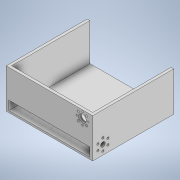
# Autodesk Inventor part: Box
Saved by Autodesk Inventor 2020.3 (Build 243373010, 373A)
## iProperties
Created: 2020-12-16
Part Number: Box
Material: Generic
Document SubType Name: Modeling
Designer: Owner
Density: 1 g/cm^3
Appearance: Default
Author: Owner
Autodesk Inventor part; units mm, degrees
ref_plane "YZ Plane" through (0, 0, 0) normal (1, 0, 0) x (0, 1, 0)
ref_plane "XZ Plane" through (0, 0, 0) normal (0, 1, 0) x (-1, 0, 0)
ref_plane "XY Plane" through (0, 0, 0) normal (0, 0, 1) x (1, 0, 0)
sketch "Sketch1" plane through (0, 0, 0) normal (0, 1, 0) x (-1, 0, 0)
  line L0 (73.3806, 68.834) -> (-73.3806, 68.834)
  line L1 (-73.3806, 68.834) -> (-73.3806, -68.834)
  line L2 (-73.3806, -68.834) -> (73.3806, -68.834)
  line L3 (73.3806, -68.834) -> (73.3806, 68.834)
  line L4 (73.3806, 68.834) -> (-73.3806, -68.834) construction
  line L5 (-73.3806, 68.834) -> (73.3806, -68.834) construction
  point P0 (0, 0)
  dimension "d0" = 146.7612
  dimension "d1" = 137.668
  constraints: 12 end point, 2 midpoint, 2 parallel, 1 horizontal, 1 perpendicular
  measures "d0" distance of L2.end L1.end
  measures "d1" distance of L1.end L0.end
extrude "Extrusion1" add sketch "Sketch1" along normal blind 3.175
sketch "Sketch2" plane through (0, 3.175, 0) normal (0, 1, 0) x (1, 0, 0)
  line L0 (73.3806, 68.834) -> (-73.3806, 68.834) projected
  line L1 (-68.834, -68.834) -> (68.834, -68.834)
  line L2 (68.834, -68.834) -> (68.834, 68.834)
  line L3 (68.834, 68.834) -> (-68.834, 68.834)
  line L4 (-68.834, 68.834) -> (-68.834, -68.834)
  line L5 (-68.834, -68.834) -> (68.834, 68.834) construction
  line L6 (68.834, -68.834) -> (-68.834, 68.834) construction
  line L7 (73.3806, -68.834) -> (73.3806, 68.834) projected
  line L8 (73.3806, 68.834) -> (68.834, 68.834)
  line L9 (68.834, 68.834) -> (68.834, -68.834)
  line L10 (68.834, -68.834) -> (73.3806, -68.834)
  line L11 (73.3806, -68.834) -> (73.3806, 68.834)
  line L12 (-73.3806, 68.834) -> (-68.834, 68.834)
  line L13 (-68.834, 68.834) -> (-68.834, -68.834)
  line L14 (-68.834, -68.834) -> (-73.3806, -68.834)
  line L15 (-73.3806, -68.834) -> (-73.3806, 68.834)
  point P0 (0, 0)
  dimension "d4" = 137.668
  constraints: 28 end point, 6 parallel, 3 horizontal, 3 perpendicular, 2 midpoint, 1 point on line
  measures "d4" distance of L3.end L2.end
extrude "Extrusion2" add sketch "Sketch2" along normal blind 63.5 contours L7 L10 L2 L0 | L4 L14 L15 L0
sketch "Sketch3" plane through (0, 3.175, 0) normal (0, 1, 0) x (1, 0, 0)
  line L0 (-68.834, -68.834) -> (68.834, -68.834) projected
  line L1 (68.834, 68.834) -> (68.834, -68.834) projected
  line L2 (-68.834, -68.834) -> (68.834, -68.834)
  line L3 (68.834, -68.834) -> (68.834, -64.2874)
  line L4 (68.834, -64.2874) -> (-68.834, -64.2874)
  line L5 (-68.834, -64.2874) -> (-68.834, -68.834)
  point P0 (0, 0)
  dimension "d7" = 4.5466
  constraints: 8 end point, 2 parallel, 1 horizontal, 1 perpendicular, 1 point on line
  measures "d7" distance of L3.end L2.end
extrude "Extrusion3" add sketch "Sketch3" along normal blind 63.5
sketch "Sketch4" plane through (-73.3806, 0, 68.834) normal (0, 0, 1) x (1, 0, 0)
  line L0 (142.2146, 3.175) -> (4.5466, 3.175) projected
  line L1 (142.2146, 3.175) -> (142.2146, 66.675) projected
  line L2 (4.5466, 3.175) -> (142.2146, 3.175)
  line L3 (142.2146, 3.175) -> (142.2146, 18.415)
  line L4 (142.2146, 18.415) -> (4.5466, 18.415)
  line L5 (4.5466, 18.415) -> (4.5466, 3.175)
  point P0 (73.3806, 0)
  dimension "d10" = 15.24
  constraints: 8 end point, 2 parallel, 1 horizontal, 1 perpendicular, 1 point on line
  measures "d10" distance of L3.end L2.end
extrude "Extrusion4" cut sketch "Sketch4" against normal blind 25.4
sketch "Sketch5" plane through (73.3806, 0, 68.834) normal (1, 0, 0) x (0, 0, -1)
  line L0 (4.5466, 66.675) -> (4.5466, 18.415) projected
  line L1 (4.5466, 20.7271) -> (4.5466, 3.175)
  line L2 (0, 3.175) -> (137.668, 3.175) projected
  line L3 (4.5466, 3.175) -> (29.9466, 3.175)
  line L4 (29.9466, 3.175) -> (29.9466, 28.575)
  line L5 (29.9466, 28.575) -> (4.5466, 28.575)
  line L6 (4.5466, 28.575) -> (4.5466, 3.175)
  circle A0 centre (17.2466, 15.875) radius 12.7
  circle A1 centre (17.2466, 15.875) radius 3.81
  line L7 (17.2466, 15.875) -> (17.2466, 25.654)
  circle A2 centre (17.2466, 25.654) radius 1.778
  circle A3 centre (8.7777, 20.7645) radius 1.778
  circle A4 centre (8.7777, 10.9855) radius 1.778
  circle A5 centre (17.2466, 6.096) radius 1.778
  circle A6 centre (25.7155, 10.9855) radius 1.778
  circle A7 centre (25.7155, 20.7645) radius 1.778
  point P0 (68.834, 0)
  dimension "d13" = 25.4
  dimension "d14" = 25.4
  dimension "d15" = 25.4
  dimension "d16" = 7.62
  dimension "d17" = 9.779
  dimension "d18" = 3.556
  dimension "d21" = 360
  constraints: 12 end point, 8 centre point, 2 coincident, 2 parallel, 2 point on line, 2 vertical, 1 horizontal, 1 perpendicular, 13 other
  measures "d13" distance of L5.end L4.end
  measures "d14" distance of L4.end L3.end
  measures "d15" diameter of A0
  measures "d16" diameter of A1
  measures "d17" distance of L7.start L7.end
  measures "d18" diameter of A2
extrude "Extrusion5" cut sketch "Sketch5" against normal blind 25.4 contours A1 | A2 | A3 | A4 | A5 | A6 | A7
sketch "Sketch6" plane through (-73.3806, 0, 68.834) normal (0, 0, 1) x (1, 0, 0)
  line L0 (142.2146, 18.415) -> (142.2146, 66.675) projected
  line L1 (142.2146, 66.675) -> (116.8146, 66.675)
  line L2 (116.8146, 66.675) -> (116.8146, 41.275)
  line L3 (116.8146, 41.275) -> (142.2146, 41.275)
  line L4 (142.2146, 41.275) -> (142.2146, 66.675)
  circle A0 centre (129.5146, 53.975) radius 6.3627
  line L5 (129.5146, 53.975) -> (129.5146, 63.754)
  circle A1 centre (129.5146, 63.754) radius 1.3589
  circle A2 centre (119.7356, 53.975) radius 1.3589
  circle A3 centre (129.5146, 44.196) radius 1.3589
  circle A4 centre (139.2936, 53.975) radius 1.3589
  line L6 (129.5146, 53.975) -> (116.8146, 66.675)
  line L7 (129.5146, 53.975) -> (122.5998, 60.8898)
  circle A5 centre (122.5998, 60.8898) radius 1.778
  circle A6 centre (122.5998, 47.0602) radius 1.778
  circle A7 centre (136.4294, 47.0602) radius 1.778
  circle A8 centre (136.4294, 60.8898) radius 1.778
  point P0 (73.3806, 0)
  dimension "d25" = 25.4
  dimension "d26" = 25.4
  dimension "d27" = 12.7254
  dimension "d28" = 9.779
  dimension "d29" = 2.7178
  dimension "d32" = 360
  dimension "d34" = 9.779
  dimension "d35" = 3.556
  dimension "d38" = 360
  constraints: 14 end point, 9 centre point, 2 coincident, 2 parallel, 1 horizontal, 1 perpendicular, 1 point on line, 1 vertical, 18 other
  measures "d25" distance of L3.end L2.end
  measures "d26" distance of L2.end L1.end
  measures "d27" diameter of A0
  measures "d28" distance of L5.start L5.end
  measures "d29" diameter of A1
  measures "d34" distance of L5.start L7.end
  measures "d35" diameter of A5
extrude "Extrusion6" cut sketch "Sketch6" against normal blind 25.4 contours A1 | A0 L5 L6 | L6 L5 A0 | A5 L6 | L6 A5 | A2 | A3 | A4 | A6 | A7 | A8
body "Solid1"
